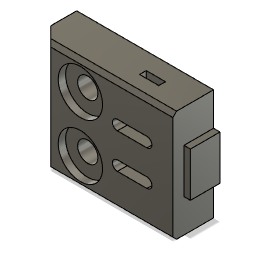
endstop_limit_switch (Autodesk Fusion 360 design; units mm, degrees)
Autodesk Fusion 360 part; units mm, degrees
sketch "Sketch1" plane through (0, 0, 0) normal (0, 0, 1) x (1, 0, 0)
  line L0 (0, 0) -> (37, 0)
  line L1 (37, 0) -> (37, 30)
  line L2 (37, 30) -> (0, 30)
  line L3 (0, 30) -> (0, 0)
  circle A0 centre (12, 22.5) radius 2.75
  circle A1 centre (12, 7.5) radius 2.75
  line L4 (12, 30) -> (12, 0) construction
  line L5 (12, 15) -> (37, 15) construction
  circle A2 centre (12, 22.5) radius 6
  circle A3 centre (12, 7.5) radius 6
  line L6 (37, 21) -> (38.75, 21)
  line L7 (38.75, 21) -> (38.75, 9)
  line L8 (38.75, 9) -> (37, 9)
  line L9 (30, 21.1) -> (22, 21.1)
  arc A4 (22, 21.1) -> (22, 18.4) centre (22, 19.75) ccw
  line L10 (22, 18.4) -> (30, 18.4)
  arc A5 (30, 18.4) -> (30, 21.1) centre (30, 19.75) ccw
  line L11 (30, 19.75) -> (22, 19.75) construction
  line L12 (30, 19.75) -> (22, 19.75) construction
  line L13 (22, 11.6) -> (30, 11.6)
  arc A6 (30, 8.9) -> (30, 11.6) centre (30, 10.25) ccw
  arc A7 (22, 11.6) -> (22, 8.9) centre (22, 10.25) ccw
  line L14 (30, 8.9) -> (22, 8.9)
  line L15 (27.5, 25) -> (37, 25) construction
  line L16 (37, 25) -> (37, 5) construction
  line L17 (37, 5) -> (27.5, 5) construction
  line L18 (27.5, 5) -> (27.5, 25) construction
  line L19 (19.4, 22.35) -> (32.6, 22.35)
  line L20 (32.6, 22.35) -> (32.6, 17.15)
  line L21 (32.6, 17.15) -> (19.4, 17.15)
  line L22 (19.4, 17.15) -> (19.4, 22.35)
  line L23 (26, 19.75) -> (26, 22.35) construction
  line L24 (22, 19.75) -> (19.4, 19.75) construction
  line L25 (32.6, 12.85) -> (19.4, 12.85)
  line L26 (19.4, 12.85) -> (19.4, 7.65)
  line L27 (32.6, 7.65) -> (32.6, 12.85)
  line L28 (19.4, 7.65) -> (32.6, 7.65)
  line L29 (23.4, 22.35) -> (23.4, 30)
  line L30 (28.6, 30) -> (28.6, 22.35)
  line L31 (23.4, 7.65) -> (23.4, 0)
  line L32 (28.6, 0) -> (28.6, 7.65)
  dimension "d1" = 15
  dimension "d2" = 5.5
  dimension "d3" = 12
  dimension "d4" = 1.75
  dimension "d5" = 12
  dimension "d14" = 2.7
  dimension "d16" = 9.5
  dimension "d17" = 30
  dimension "d19" = 8
  dimension "d20" = 7
  dimension "d22" = 9.5
  dimension "d23" = 20
  dimension "d24" = 10
  dimension "d25" = 12
  dimension "d26" = 5.2
  dimension "d27" = 2.6
  dimension "d28" = 5.2
  constraint horizontal L0
  constraint vertical L1
  constraint horizontal L2
  constraint vertical L3
  constraint coincident L0.start L3.end
  constraint coincident L2 L4.start
  constraint coincident L0 L4.end
  constraint perpendicular L0 L4
  constraint coincident A1.centre L4
  constraint coincident A0.centre L4
  constraint midpoint L1 L5.end
  constraint perpendicular L1 L5
  constraint midpoint L4 L5.start
  constraint symmetric A0 A1 L5
  constraint concentric A0 A2
  constraint concentric A1 A3
  constraint equal A2 A3
  constraint coincident L1 L6.start
  constraint perpendicular L1 L6
  constraint perpendicular L6 L7
  constraint coincident L1 L8.end
  constraint perpendicular L1 L8
  constraint symmetric L5 L6 L8
  constraint tangent L9 A4
  constraint tangent A4 L10
  constraint parallel L9 L10
  constraint tangent L10 A5
  constraint tangent L9 A5
  constraint parallel L2 L11
  constraint coincident A4.centre L11.end
  constraint parallel L11 L12
  constraint coincident A5.centre L11.start
  constraint symmetric L5 L9.start A6.start
  constraint symmetric L5 L9.end A7.end
  constraint symmetric L5 A4.end L13.start
  constraint symmetric L5 L10.end L13.end
  constraint symmetric L5 A4 A7
  constraint symmetric L5 A5 A6
  constraint horizontal L15
  constraint vertical L16
  constraint horizontal L17
  constraint vertical L18
  constraint symmetric L5 L15 L17
  constraint coincident L1 L15.end
  constraint horizontal L19
  constraint vertical L20
  constraint horizontal L21
  constraint vertical L22
  constraint symmetric L12 L19 L21
  constraint midpoint L11 L23.start
  constraint midpoint L19 L23.end
  constraint perpendicular L19 L23
  constraint perpendicular L22 L24
  constraint midpoint L22 L24.end
  constraint symmetric L5 L19.start L26.end
  constraint symmetric L5 L19.end L27.start
  constraint symmetric L5 L20.end L25.start
  constraint symmetric L5 L21.end L25.end
  constraint coincident L19 L29.start
  constraint coincident L2 L29.end
  constraint perpendicular L2 L29
  constraint coincident L2 L30.start
  constraint coincident L19 L30.end
  constraint perpendicular L19 L30
  constraint symmetric L23 L29 L30
  constraint symmetric L5 L29.start L31.start
  constraint symmetric L5 L29.end L31.end
  constraint symmetric L5 L30.start L32.start
  constraint symmetric L5 L30.end L32.end
  measures "d1" distance of A0.centre A1.centre
  measures "d2" diameter of A0
  measures "d3" diameter of A2
  measures "d4" distance of L6.start L6.end
  measures "d5" distance of L6.end L7.end
  measures "d14" diameter of A4
  measures "d16" distance of A5.centre A6.centre
  measures "d17" distance of L0.start L2.end
  measures "d19" distance of A5.centre A4.centre
  measures "d20" distance of A5.centre L16
  measures "d22" distance of L15.start L15.end
  measures "d23" distance of L15.end L16.end
  measures "d24" distance of L4 A4.centre
  measures "d25" distance of L3 L4
  measures "d26" distance of L19.end L20.end
  measures "d27" distance of A4.centre L24.end
  measures "d28" distance of L29 L30
extrude "Extrude1" add sketch "Sketch1" along normal blind 11 contours L0 L1 L2 L3 L19 L20 L21 L22 L25 L26 L27 L28 L29 L30 L31 L32 | L0 L28 L31 L32 | L25 L26 L27 L28 | L2 L19 L29 L30 | L19 L20 L21 L22 | A2 | A3
extrude "Extrude2" add sketch "Sketch1" along normal blind 8 contours L1 L6 L7 L8
extrude "Extrude3" cut sketch "Sketch1" against normal blind 2 from surface at 11 contours A2 | A3
chamfer "Chamfer2" distance 1 angle 45 2 edges at (18.5, 0, 11) (18.5, 30, 11)
chamfer "Chamfer1" distance 4 angle 45 1 edges at (0, 15, 11)
ref_plane "WorkPlane1" through (18.5, 15, 5.5) normal (0, 0, 1) x (1, 0, 0)
extrude "Extrude4" cut sketch "Sketch1" along normal mid plane 1.8 from surface at 5.5 contours L0 L28 L31 L32 | L25 L26 L27 L28 | L2 L19 L29 L30 | L19 L20 L21 L22
extrude "Extrude5" add sketch "Sketch1" along normal blind 0.2 from surface at 6.4 contours L9 A4 L10 A5 | L13 A6 A7 L14
equation "d27 = d26 / 2"
equation "d28 = d26"
